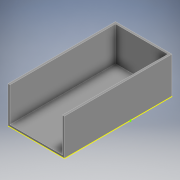
# Autodesk Inventor part: Part1
Saved by Autodesk Inventor 2021 (Build 250183000, 183)
## iProperties
Created: 2023-01-12
Part Number: Part1
Material: Generic
Document SubType Name: Modeling
Designer: boyle
Density: 1 g/cm^3
Appearance: Default
Author: boyle
Autodesk Inventor part; units mm, degrees
ref_plane "YZ Plane" through (0, 0, 0) normal (1, 0, 0) x (0, 1, 0)
ref_plane "XZ Plane" through (0, 0, 0) normal (0, 1, 0) x (-1, 0, 0)
ref_plane "XY Plane" through (0, 0, 0) normal (0, 0, 1) x (1, 0, 0)
sketch "Sketch1" plane through (0, 0, 0) normal (0, 1, 0) x (-1, 0, 0)
  line L0 (0, 0) -> (-107.95, 0)
  line L1 (-107.95, 0) -> (-107.95, 209.55)
  line L2 (-107.95, 209.55) -> (0, 209.55)
  line L3 (0, 209.55) -> (0, 0)
  dimension "d0" = 107.95
  dimension "d1" = 209.55
  constraints: 8 end point, 2 parallel, 1 horizontal, 1 perpendicular
  measures "d0" distance of L1.end L2.end
  measures "d1" distance of L0.end L1.end
extrude "Extrusion1" add sketch "Sketch1" along normal blind 69.85
shell "Shell1" thickness 3.81 removed faces 1 at (35.9833, 69.85, 69.85)
sketch "Sketch2" plane through (0, 0, 209.55) normal (0, 0, 1) x (1, 0, 0)
  line L0 (0, 0) -> (107.95, 0) projected
  line L1 (107.95, 0) -> (107.95, 69.85) projected
  line L2 (0, 69.85) -> (107.95, 69.85) projected
  line L3 (0, 0) -> (0, 69.85) projected
  point P0 (0, 0)
extrude "Extrusion2" cut sketch "Sketch2" against normal up to surface (3.81 mm away)
sketch "Sketch3" plane through (0, 0, 0) normal (0, -1, 0) x (1, 0, 0)
  line L0 (107.95, 205.74) -> (0, 205.74) projected
  line L1 (0, 0) -> (0, 205.74) projected
  line L2 (107.95, 205.74) -> (107.95, 0) projected
  line L3 (107.95, 205.74) -> (0, 205.74) projected
  line L4 (0, 0) -> (0, 205.74) projected
  line L5 (107.95, 0) -> (0, 0) projected
  line L6 (107.95, 205.74) -> (107.95, 0) projected
  line L7 (107.95, 205.74) -> (107.95, 0) projected
  line L8 (0, 0) -> (0, 205.74) projected
  spline S0 degree 4 poles (107.95, 80.2566) (92.1768, 134.9496) (63.3079, -17.6427) (18.0672, 199.1019) (14.9699, 60.2362) (0, 102.87) knots 0 0 0 0 0 0.533001 1 1 1 1 1
  point P0 (82.9333, 90.6004)
  point P1 (54.9148, 82.3829)
  point P2 (27.0432, 107.7403)
  point P3 (14.461, 94.2963)
  point P4 (0, 102.87)
  point P5 (107.95, 80.2566)
  constraints: 1 midpoint, 1 point on line, 6 other
body "Solid1"
